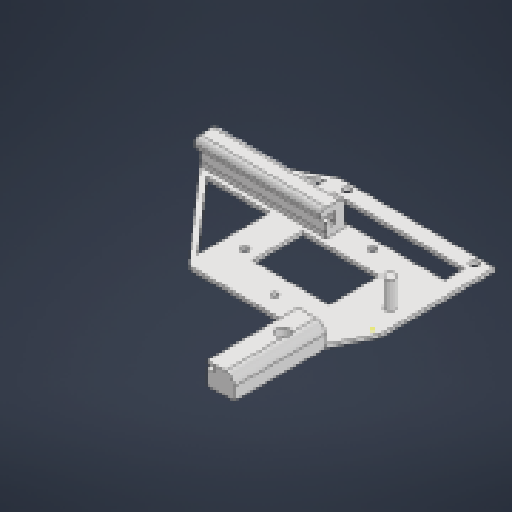
# Autodesk Inventor part: BasePlate
Saved by Autodesk Inventor 2026.1 (Build 301233020, 233B)
## iProperties
Created: 2025-10-14
Part Number: BasePlate
Material: Generic
Document SubType Name: Modeling
Designer: alexj
Density: 1 g/cm^3
Appearance: Default
Mass: 32.0674 g
Surface Area: 273.946 cm^2
Volume: 32.0674 cm^3
Author: alexj
Autodesk Inventor part; units mm, degrees
ref_plane "YZ Plane" through (0, 0, 0) normal (1, 0, 0) x (0, 1, 0)
ref_plane "XZ Plane" through (0, 0, 0) normal (0, 1, 0) x (-1, 0, 0)
ref_plane "XY Plane" through (0, 0, 0) normal (0, 0, 1) x (1, 0, 0)
sketch "Sketch1" plane through (0, 0, 0) normal (0, 1, 0) x (-1, 0, 0)
  line L0 (125, 0) -> (125, -63)
  line L1 (125, -63) -> (-4.2, -63)
  line L2 (-4.2, -63) -> (-4.2, 0)
  line L3 (-4.2, 0) -> (5.8, 0)
  line L4 (5.8, 0) -> (5.8, 40)
  line L5 (20.8, 40) -> (20.8, 0)
  line L6 (20.8, 0) -> (125, 0)
  line L7 (5.8, 40) -> (5.8, 70)
  line L8 (5.8, 70) -> (20.8, 70)
  line L9 (20.8, 70) -> (20.8, 40)
  line L10 (125, 0) -> (125, 20)
  line L11 (125, 20) -> (5.8, 20)
  line L12 (-4.2, -1.8) -> (-4.2, -60.8) projected
  line L13 (-4.2, 0) -> (5.8, 20)
  line L14 (125, -35.426) -> (125, -25.426) projected
  point P0 (20.8, 20)
  dimension "d1" = 63
  dimension "d2" = 15
  dimension "d3" = 40
  dimension "d4" = 10
  dimension "d51" = 30
  dimension "d127" = 20
  dimension "d129" = 126.9309
  dimension "d130" = 104.2
  dimension "d131" = 13.4164
  constraints: 26 end point, 6 perpendicular, 3 point on line, 3 vertical, 2 parallel, 1 collinear, 1 horizontal, 1 midpoint
  measures "d1" distance of L1.end L2.end
  measures "d2" distance of L4.end L5.start
  measures "d3" distance of L3.end L4.end
  measures "d4" distance of L2.end L3.end
  measures "d51" distance of L5.start L8.end
  measures "d127" distance between parallel lines of L11 L6
  measures "d129" distance from line of L14.end L13
  measures "d130" distance from line of point (20.8, 20) L14
  measures "d131" distance from line of point (20.8, 20) L13
extrude "Extrusion1" add sketch "Sketch1" along normal blind 2
sketch "Sketch2" plane through (0, 2, 0) normal (0, 1, 0) x (1, 0, 0)
  line L0 (-73.3, 3.3) -> (-3.3, 3.3) construction
  line L1 (-3.3, 3.3) -> (-3.3, 59.3) construction
  line L2 (-3.3, 59.3) -> (-73.3, 59.3) construction
  line L3 (-73.3, 59.3) -> (-73.3, 3.3) construction
  circle A0 centre (-73.3, 3.3) radius 1.7
  circle A1 centre (-73.3, 59.3) radius 1.7
  circle A2 centre (-3.3, 59.3) radius 1.7
  point P0 (0, 0)
  dimension "d7" = 70
  dimension "d8" = 56
  dimension "d9" = 3.3
  dimension "d11" = 3.4
  dimension "d12" = 3.4
  dimension "d13" = 3.4
  dimension "d197" = 3.3
  constraints: 8 end point, 3 centre point, 3 coincident, 2 parallel, 1 horizontal, 1 perpendicular
  measures "d7" distance of L2.end L1.end
  measures "d8" distance of L0.end L1.end
  measures "d9" distance from line of point (0, 0) L1
  measures "d11" diameter of A0
  measures "d12" diameter of A1
  measures "d13" diameter of A2
  measures "d197" horizontal distance of point (0, 0) L0.end
hole "Hole1" at (-73.3, 2, -3.3) at (-73.3, 2, -59.3) at (-3.3, 2, -59.3) direction (0, -1, 0) diameter 4.4 end through all
sketch "Sketch3" plane through (0, 2, 0) normal (0, 1, 0) x (1, 0, 0)
  circle A0 centre (-3.3, 59.3) radius 2.2 construction
  circle A1 centre (-73.3, 59.3) radius 2.2 construction
  circle A2 centre (-73.3, 3.3) radius 2.2 construction
  line L0 (-20.8, -20) -> (-20.8, -70) construction
  line L1 (-5.8, -70) -> (-5.8, -20) construction
  line L2 (4.2, 0) -> (4.2, 63) construction
  line L3 (4.2, 63) -> (-125, 63) construction
  line L4 (-73.3, 3.3) -> (-3.3, 3.3) construction
  line L5 (-3.3, 3.3) -> (-3.3, 59.3) construction
  line L6 (-3.3, 38.3) -> (-38.3, 38.3) construction
  line L7 (-38.3, 38.3) -> (-38.3, 3.3) construction
  circle A3 centre (-38.3, 38.3) radius 2.2 construction
  line L8 (-20.8, -70) -> (-5.8, -70) projected
  line L9 (-5.8, -20) -> (4.2, 0) projected
  line L10 (-125, 63) -> (-125, -20) projected
  line L11 (-125, -20) -> (-20.8, -20) projected
  point P0 (0, 0)
  dimension "d24" = 35
  dimension "d25" = 35
  dimension "d26" = 4.4
  constraints: 8 end point, 2 horizontal, 2 perpendicular, 1 centre point, 1 coincident, 1 midpoint, 1 point on line
  measures "d24" distance of L6.start L6.end
  measures "d25" distance of L6.end L7.end
  measures "d26" diameter of A3
hole "Hole2" at (-38.3, 2, -38.3) direction (0, -1, 0) diameter 4.4 end through all
sketch "Sketch5" plane through (0, 2, 0) normal (0, 1, 0) x (1, 0, 0)
  circle A0 centre (-38.3, 38.3) radius 2.2 projected
  circle A1 centre (-5.5339, 15.3569) radius 2.625
  line L0 (-38.3, 38.3) -> (-5.5339, 15.3569)
  line L1 (-38.3, 38.3) -> (-38.3, 10.8789)
  point P0 (0, 0)
  dimension "d44" = 5.25
  dimension "d46" = 40
  dimension "d47" = 55
  dimension "d200" = 27.4211
  constraints: 4 end point, 1 centre point, 1 vertical
  measures "d44" diameter of A1
  measures "d46" distance of L0.start L0.end
  measures "d47" angle of L0 L1
  measures "d200" distance of L0.start L1.end
extrude "Extrusion2" add sketch "Sketch5" along normal blind 15 contours A1
sketch "Sketch6" plane through (0, 2, 0) normal (0, 1, 0) x (1, 0, 0)
  line L0 (-80.8, 40.4259) -> (-55.8, 40.4259)
  line L1 (-55.8, 40.4259) -> (-55.8, 30.4259)
  line L2 (-55.8, 30.4259) -> (-80.8, 30.4259)
  line L3 (-80.8, 30.4259) -> (-80.8, 40.4259)
  circle A0 centre (-5.5339, 15.3569) radius 2.625 projected
  circle A1 centre (-5.5339, 15.3569) radius 2.625 projected
  line L4 (-5.5339, 15.3569) -> (-80.8, 15.3569) construction
  point P0 (0, 0)
  point P1 (-55.8, 35.4259)
  dimension "d54" = 10
  dimension "d132" = 25
  dimension "d133" = 30.4259
  dimension "d134" = 66.0957
  dimension "d206" = 80.8
  constraints: 10 end point, 2 horizontal, 2 parallel, 1 midpoint, 1 perpendicular
  measures "d54" distance of L2.end L0.start
  measures "d132" distance of L1.end L2.end
  measures "d133" distance from line of point (0, 0) L2
  measures "d134" distance of point (-55.8, 35.426) point (0, 0)
  measures "d206" horizontal distance of point (0, 0) L4.end
extrude "Extrusion3" add sketch "Sketch6" along normal blind 15 contours L0 L1 L2 L3
sketch "Sketch7" plane through (-80.8, 2, -40.4259) normal (-1, 0, 0) x (0, 0, 1)
  line L0 (10, 2.5) -> (5, 2.5)
  line L1 (9.9999, 7.5) -> (6.9999, 7.5) projected
  line L2 (10, 0) -> (10, 15) projected
  line L3 (4.9999, 5) -> (6.9999, 5) projected
  line L4 (6.9999, 5) -> (6.9999, 7.5) projected
  line L5 (-22.5741, 0) -> (60.4259, 0) projected
  line L6 (7.2499, 7.5) -> (7.2499, 5)
  line L7 (7.2499, 5) -> (6.9999, 5)
  line L8 (5, 10.45) -> (10, 10.45)
  line L9 (5, 10.45) -> (5, 2.5)
  line L10 (7.2499, 7.5) -> (9.9999, 7.5)
  line L11 (10, 2.5) -> (9.9999, 7.5)
  point P0 (5, 5)
  dimension "d186" = 0.25
  dimension "d256" = 2.5
  dimension "d257" = 0.25
  dimension "d274" = 7.95
  dimension "d275" = 5
  constraints: 14 end point, 3 point on line, 2 perpendicular, 2 vertical, 1 horizontal
  measures "d186" distance between parallel lines of L6 L4
  measures "d256" distance between parallel lines of L5 L0
  measures "d257" distance of L6.end L3.end
  measures "d274" distance of L8.start L0.end
  measures "d275" distance of L8.start L8.end
extrude "Extrusion4" cut sketch "Sketch7" against normal up to surface (25 mm away) contours L1 L4 L3 L9 L8 L2 | L6 L7 L4 L1
sketch "Sketch13" plane through (0, 2, 0) normal (0, 1, 0) x (1, 0, 0)
  point P0 (0, 0)
sketch "Sketch15" plane through (-80.8, 2, -40.4259) normal (-1, 0, 0) x (0, 0, 1)
  line L0 (10, 10.45) -> (10, 15) projected
  line L1 (0, 15) -> (10, 15) projected
  line L2 (0, 0) -> (0, 15) projected
  line L3 (10, 0) -> (0, 0) projected
  line L4 (10, 0) -> (10, 2.5) projected
  line L5 (5, 10.45) -> (10, 10.45) projected
  line L6 (5, 5) -> (5, 10.45) projected
  line L7 (10, 2.5) -> (9.9999, 7.5) projected
  line L8 (9.9999, 7.5) -> (7.2499, 7.5) projected
  line L9 (7.2499, 7.5) -> (7.2499, 5) projected
  line L10 (7.2499, 5) -> (5, 5) projected
  point P0 (40.4259, -2)
extrude "Extrusion9" add sketch "Sketch15" along normal up to surface (44.2 mm away)
sketch "Sketch18" plane through (0, 2, 0) normal (0, 1, 0) x (1, 0, 0)
  point P0 (0, 0)
  point P1 (-43.3, -10.4414)
  point P2 (-13.3, -35.9207)
hole "Hole4" at (-43.3, 2, 10.4414) at (-13.3, 2, 35.9207) direction (0, -1, 0) diameter 3.4 end through all
chamfer "Chamfer1" distance 50.5 distance2 44.25 1 edges at (-125, 1, 20) measured on face at (-125, 0.6667, -24.4753)
chamfer "Chamfer2" distance 44.25 distance2 22.5 1 edges at (-125, 1, -63) measured on face at (-38.8667, 1.3333, -63)
sketch "Sketch19" plane through (0, 2, 0) normal (0, 1, 0) x (1, 0, 0)
  line L0 (-125, 30.5) -> (-80.75, -20) projected
  line L1 (-80.75, -20) -> (-80.75, 30.4259)
  line L2 (-55.8, 30.4259) -> (-124.9351, 30.4259) projected
  line L3 (-124.9351, 30.4259) -> (-80.75, -20)
  line L4 (-80.75, 63.1491) -> (-125, 40.4259)
  line L5 (-125, 40.4259) -> (-80.75, 40.4259)
  line L6 (-80.75, 40.4259) -> (-80.75, 63.1491)
  line L7 (-80.75, 30.4259) -> (-124.9351, 30.4259)
  line L8 (-83.75, 27.4259) -> (-83.75, -12.0241)
  line L9 (-83.75, -12.0241) -> (-118.3176, 27.4259)
  line L10 (-118.3176, 27.4259) -> (-83.75, 27.4259)
  line L11 (-83.75, 43.4259) -> (-112.5906, 43.4259)
  line L12 (-112.5906, 43.4259) -> (-83.75, 58.2361)
  line L13 (-83.75, 58.2361) -> (-83.75, 43.4259)
  line L14 (-80.75, 0) -> (-20.75, 0)
  line L15 (-20.75, 0) -> (-20.75, 30.4259)
  line L16 (-20.75, 30.4259) -> (-80.75, 30.4259)
  line L17 (-80.75, 0) -> (-80.75, 30.4259)
  line L18 (-80.75, 27.4259) -> (-23.75, 27.4259)
  line L19 (-23.75, 27.4259) -> (-23.75, 0)
  line L20 (-65.85, 0) -> (-65.85, 27.4259)
  circle A0 centre (-73.3, 3.3) radius 2.2 projected
  line L21 (-75.75, 54.3) -> (-3.8, 54.3)
  line L22 (-3.8, 54.3) -> (-3.8, 43.3)
  line L23 (-3.8, 43.3) -> (-75.75, 43.3)
  line L24 (-75.75, 43.3) -> (-75.75, 54.3)
  line L25 (4.2, 0) -> (4.2, 63) projected
  circle A1 centre (-38.3, 38.3) radius 2.2 projected
  circle A2 centre (-73.3, 59.3) radius 2.9111 projected
  point P0 (0, 0)
  dimension "d160" = 3
  dimension "d161" = 3
  dimension "d164" = 60
  dimension "d165" = 30.4259
  dimension "d167" = 3
  dimension "d168" = 3
  dimension "d169" = 7.45
  dimension "d176" = 5
  dimension "d177" = 8
  dimension "d178" = 5
  dimension "d179" = 5
  dimension "d312" = 49.7434
  constraints: 46 end point, 10 perpendicular, 8 point on line, 2 horizontal, 2 parallel, 1 collinear, 1 vertical, 4 other
  measures "d160" distance between parallel lines of L1 L8
  measures "d161" distance between parallel lines of L5 L11
  measures "d164" distance of L14.start L14.end
  measures "d165" distance between parallel lines of L2 L14
  measures "d167" distance between parallel lines of L15 L19
  measures "d168" distance between parallel lines of L16 L18
  measures "d169" distance from line of L20 A0.centre
  measures "d176" distance between parallel lines of L24 L6
  measures "d177" distance between parallel lines of L25 L22
  measures "d178" distance from line of A2.centre L21
  measures "d179" distance from line of L23 A1.centre
  measures "d312" distance of L4.start L4.end
extrude "Extrusion11" cut sketch "Sketch19" against normal blind 10 contours L20 L18 L19 L14 | L8 L9 L10 | L11 L12 L13 | L21 L22 L23 L24
sketch "Sketch20" plane through (-125, 17, -30.4259) normal (0, 0, 1) x (1, 0, 0)
  line L0 (0, -4.55) -> (69.2, -4.55) projected
  line L1 (69.2, -4.55) -> (69.2, 0) projected
  line L2 (69.2, 0) -> (0, 0) projected
  line L3 (0, 0) -> (0, -4.55) projected
  point P0 (125, -17)
extrude "Extrusion12" add sketch "Sketch20" along normal blind 3
fillet "Fillet1" radius 3 2 edges at (-90.4, 17, -40.4259) (-90.4, 17, -27.4259)
sketch "Sketch21" plane through (0, 2, 0) normal (0, 1, 0) x (1, 0, 0)
  line L0 (-80.75, -20) -> (-20.8, -20) projected
  line L1 (-20.8, -70) -> (-5.8, -70) projected
  line L2 (-20.8, -20) -> (-5.8, -20)
  line L3 (-5.8, -20) -> (-5.8, -70)
  line L4 (-5.8, -70) -> (-20.8, -70)
  line L5 (-20.8, -70) -> (-20.8, -20)
  circle A0 centre (-13.3, -35.9207) radius 1.7 projected
  point P0 (0, 0)
  constraints: 8 end point, 2 parallel, 1 horizontal, 1 perpendicular
extrude "Extrusion13" add sketch "Sketch21" along normal blind 10
fillet "Fillet2" radius 5 1 edges at (-5.8, 12, 45)
sketch "Sketch22" plane through (-20.8, 0, 70) normal (0, 0, 1) x (1, 0, 0)
  line L0 (0, 8.6171) -> (3.5, 8)
  line L1 (3.5, 11) -> (0, 10.3829)
  line L2 (3.5, 11) -> (3.5, 8)
  line L3 (0, 0) -> (15, 0) projected
  line L4 (0, 0) -> (0, 12) projected
  line L5 (0, 10.3829) -> (0, 8.6171)
  dimension "d333" = 80
  dimension "d334" = 80
  dimension "d336" = 3
  dimension "d346" = 15
  dimension "d347" = 3.5
  dimension "d348" = 8.6171
  constraints: 8 end point, 1 equal length, 1 parallel
  measures "d333" angle of L2 L0
  measures "d334" angle of L2 L1
  measures "d336" distance of L1.start L0.end
  measures "d346" distance from line of L3.end L5
  measures "d347" distance between parallel lines of L2 L4
  measures "d348" distance of L3.start L0.start
extrude "Extrusion14" cut sketch "Sketch22" against normal blind 45
sketch "Sketch23" plane through (0, 12, 0) normal (0, 1, 0) x (1, 0, 0)
  circle A0 centre (-13.3, -35.9207) radius 1.7 projected
  point P0 (0, 0)
  constraints: 1 coincident
hole "Hole5" at (-13.3, 12, 35.9207) direction (0, -1, 0) diameter 7 depth 6
body "Solid1"
